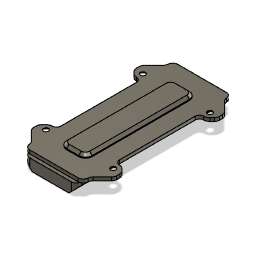
Controller Cooler (P2) [(M)SPPS000000003.2] v2 (Autodesk Fusion 360 design; units mm, degrees)
Autodesk Fusion 360 part; units mm, degrees
sketch "Sketch1" plane through (0, 0, 0) normal (0, 1, 0) x (1, 0, 0)
  line L0 (15.75, 46.1) -> (15.75, -46.1)
  line L1 (-15.75, -46.1) -> (-15.75, 46.1)
  line L2 (-15.75, -46.1) -> (15.75, -46.1)
  line L3 (-15.75, 46.1) -> (15.75, 46.1)
  line L4 (15.25, 45.6) -> (15.25, -45.6)
  line L5 (-15.25, -45.6) -> (15.25, -45.6)
  line L6 (-15.25, -45.6) -> (-15.25, 45.6)
  line L7 (-15.25, 45.6) -> (15.25, 45.6)
  circle A0 centre (19.75, 28.5) radius 3.5
  circle A1 centre (19.75, 28.5) radius 1.5
  circle A2 centre (19.75, -28.5) radius 3.5
  circle A3 centre (19.75, -28.5) radius 1.5
  circle A4 centre (-19.75, 28.5) radius 3.5
  circle A5 centre (-19.75, 28.5) radius 1.5
  circle A6 centre (-19.75, -28.5) radius 3.5
  circle A7 centre (-19.75, -28.5) radius 1.5
  line L8 (-17.25, 47.6) -> (-17.25, 39.6)
  line L9 (-17.25, 39.6) -> (-24.5, 32.35)
  line L10 (-24.5, 28.05) -> (-24.5, 32.35)
  line L11 (-16.9, 20.45) -> (-24.5, 28.05)
  line L12 (-16.9, -20.45) -> (-24.5, -28.05)
  line L13 (-24.5, -28.05) -> (-24.5, -32.35)
  line L14 (-24.5, -32.35) -> (-17.25, -39.6)
  line L15 (-17.25, -39.6) -> (-17.25, -47.6)
  line L16 (17.25, -47.6) -> (17.25, -39.6)
  line L17 (17.25, -39.6) -> (24.5, -32.35)
  line L18 (24.5, -28.05) -> (24.5, -32.35)
  line L19 (16.9, -20.45) -> (24.5, -28.05)
  line L20 (16.9, 20.45) -> (24.5, 28.05)
  line L21 (24.5, 28.05) -> (24.5, 32.35)
  line L22 (24.5, 32.35) -> (17.25, 39.6)
  line L23 (17.25, 39.6) -> (17.25, 47.6)
  line L24 (-17.25, 22.323) -> (-17.25, -22.323)
  line L25 (17.25, -22.323) -> (17.25, 22.323)
  line L26 (-17.25, 47.6) -> (17.25, 47.6)
  line L27 (-17.25, -47.6) -> (17.25, -47.6)
  arc A8 (-22.35, 25.9) -> (-19.75, 24.823) centre (-19.75, 28.5) ccw
  arc A9 (19.75, 24.823) -> (22.35, 25.9) centre (19.75, 28.5) ccw
  arc A10 (-19.75, -24.823) -> (-22.35, -25.9) centre (-19.75, -28.5) ccw
  arc A11 (22.35, -25.9) -> (19.75, -24.823) centre (19.75, -28.5) ccw
  arc A12 (17.25, -22.323) -> (19.75, -24.823) centre (19.75, -22.323) ccw
  arc A13 (-19.75, -24.823) -> (-17.25, -22.323) centre (-19.75, -22.323) ccw
  arc A14 (-17.25, 22.323) -> (-19.75, 24.823) centre (-19.75, 22.323) ccw
  arc A15 (19.75, 24.823) -> (17.25, 22.323) centre (19.75, 22.323) ccw
  dimension "d7" = 31.5
  dimension "d8" = 15.75
  dimension "d99" = -0.5
  dimension "d1586" = 7
  dimension "d1613" = 7
  dimension "d1614" = 7
  dimension "d44" = 7
  dimension "d146" = 3
  dimension "d147" = 3
  dimension "d65" = 3
  dimension "d66" = 3
  dimension "d156" = 1.5
  dimension "d157" = 19.75
  dimension "d158" = 28.5
  dimension "d159" = 28.5
  dimension "d160" = 19.75
  dimension "d161" = 92.2
  dimension "d162" = 46.1
  dimension "d163" = 1.5
  dimension "d164" = 1.5
  dimension "d167" = 1.5
  dimension "d168" = 4.3
  dimension "d169" = 4.3
  dimension "d170" = 4.3
  dimension "d171" = 4.3
  dimension "d172" = 8
  dimension "d173" = 8
  dimension "d174" = 8
  dimension "d175" = 8
  dimension "d176" = 45
  dimension "d177" = 45
  dimension "d178" = 45
  dimension "d179" = 45
  dimension "d180" = 45
  dimension "d181" = 45
  dimension "d182" = 45
  dimension "d183" = 45
  dimension "d185" = 39.5
  dimension "d186" = 4.75
  dimension "d188" = 4.75
  dimension "d197" = 2.5
  dimension "d198" = 2.5
  dimension "d199" = 2.5
  dimension "d200" = 2.5
  constraint vertical L0
  constraint vertical L1
  constraint perpendicular L0 L2
  constraint perpendicular L0 L3
  constraint vertical A2.centre A0.centre
  constraint vertical A4.centre A6.centre
  constraint concentric A4 A5
  constraint concentric A0 A1
  constraint concentric A6 A7
  constraint concentric A2 A3
  constraint horizontal A4.centre A0.centre
  constraint horizontal A2.centre A6.centre
  constraint vertical L10
  constraint vertical L21
  constraint collinear L10 L13
  constraint collinear L18 L21
  constraint collinear L8 L24
  constraint collinear L15 L24
  constraint collinear L16 L25
  constraint collinear L23 L25
  constraint concentric A7 A10
  constraint tangent L12 A10
  constraint concentric A5 A8
  constraint tangent L11 A8
  constraint concentric A3 A11
  constraint tangent L19 A11
  constraint concentric A1 A9
  constraint tangent L20 A9
  constraint coincident L11 A8.start
  constraint coincident L20 A9.end
  constraint coincident L12 A10.end
  constraint coincident L19 A11.start
  constraint tangent A11 A12
  constraint tangent L25 A12
  constraint tangent A10 A13
  constraint tangent L24 A13
  constraint tangent A8 A14
  constraint tangent L24 A14
  constraint tangent A9 A15
  constraint tangent L25 A15
  measures "d7" distance of L0 L1
  measures "d8" distance of origin L1
  measures "d1586" diameter of A2
  measures "d1613" diameter of A0
  measures "d1614" diameter of A6
  measures "d44" diameter of A4
  measures "d146" diameter of A5
  measures "d147" diameter of A1
  measures "d65" diameter of A7
  measures "d66" diameter of A3
  measures "d156" distance of L0 L25
  measures "d157" horizontal distance of origin A4.centre
  measures "d158" vertical distance of origin A4.centre
  measures "d159" vertical distance of origin A6.centre
  measures "d160" horizontal distance of origin A0.centre
  measures "d161" distance of L2 L3
  measures "d162" distance of origin L3
  measures "d163" distance of L3 L26
  measures "d164" distance of L2 L27
  measures "d167" distance of L1 L24
  measures "d168" distance of L20.end L21.end
  measures "d169" distance of L9.end L10.start
  measures "d170" distance of L12.end L13.end
  measures "d171" distance of L17.end L18.start
  measures "d172" distance of L8.end L8.start
  measures "d173" distance of L22.end L23.end
  measures "d174" distance of L16.end L16.start
  measures "d175" distance of L14.end L15.end
  measures "d176" angle of L16 L17
  measures "d177" angle of L19 L25
  measures "d178" angle of L12 L24
  measures "d179" angle of L14 L15
  measures "d180" angle of L8 L9
  measures "d181" angle of L11 L24
  measures "d182" angle of L20 L25
  measures "d183" angle of L22 L23
  measures "d185" distance of A4.centre A0.centre
  measures "d186" distance of A0.centre L21
  measures "d188" distance of A4.centre L10
  measures "d197" radius of A12
  measures "d198" radius of A13
  measures "d199" radius of A14
  measures "d200" radius of A15
extrude "Extrude1" add sketch "Sketch1" against normal blind 2 contours L4 L5 L6 L7
extrude "Extrude2" add sketch "Sketch1" along normal blind 2 contours L0 L1 L2 L3 | L4 L5 L6 L7 | A0 | A2 | A4 | A6 | L8 L9 L10 L11 L12 L13 L14 L15 L16 L17 L18 L19 L20 L21 L22 L23 L24 L25 L26 L27 A8 A9 A10 A11 A12 A13 A14 A15
chamfer "Chamfer1" distance 2 angle 45 4 edges at (18.3515, 0, 27.9576) (18.3515, 0, -29.0424) (-21.1485, 0, -29.0424) (-21.1485, 0, 27.9576)
sketch "Sketch4" plane through (0, -2, 0) normal (0, -1, 0) x (1, 0, 0)
  line L0 (15.75, -45) -> (-15.75, -45)
  line L1 (15.75, -42) -> (-15.75, -42)
  line L2 (15.75, -37) -> (-15.75, -37)
  line L3 (15.75, -44) -> (-15.75, -44)
  line L4 (-15.75, -44) -> (-15.75, -46)
  line L5 (-15.75, -46) -> (15.75, -46)
  line L6 (15.75, -46) -> (15.75, -44)
  line L7 (15.75, -38) -> (-15.75, -38)
  line L8 (-15.75, -38) -> (-15.75, -40)
  line L9 (-15.75, -40) -> (15.75, -40)
  line L10 (15.75, -40) -> (15.75, -38)
  line L11 (15.75, -32) -> (-15.75, -32)
  line L12 (-15.75, -32) -> (-15.75, -34)
  line L13 (-15.75, -34) -> (15.75, -34)
  line L14 (15.75, -34) -> (15.75, -32)
  line L15 (15.75, -26) -> (-15.75, -26)
  line L16 (-15.75, -26) -> (-15.75, -28)
  line L17 (-15.75, -28) -> (15.75, -28)
  line L18 (15.75, -28) -> (15.75, -26)
  line L19 (15.75, -20) -> (-15.75, -20)
  line L20 (-15.75, -20) -> (-15.75, -22)
  line L21 (-15.75, -22) -> (15.75, -22)
  line L22 (15.75, -22) -> (15.75, -20)
  line L23 (15.75, -14) -> (-15.75, -14)
  line L24 (-15.75, -14) -> (-15.75, -16)
  line L25 (-15.75, -16) -> (15.75, -16)
  line L26 (15.75, -16) -> (15.75, -14)
  line L27 (15.75, -8) -> (-15.75, -8)
  line L28 (-15.75, -8) -> (-15.75, -10)
  line L29 (-15.75, -10) -> (15.75, -10)
  line L30 (15.75, -10) -> (15.75, -8)
  line L31 (15.75, -2) -> (-15.75, -2)
  line L32 (-15.75, -2) -> (-15.75, -4)
  line L33 (-15.75, -4) -> (15.75, -4)
  line L34 (15.75, -4) -> (15.75, -2)
  line L35 (15.75, 4) -> (-15.75, 4)
  line L36 (-15.75, 4) -> (-15.75, 2)
  line L37 (-15.75, 2) -> (15.75, 2)
  line L38 (15.75, 2) -> (15.75, 4)
  line L39 (15.75, 10) -> (-15.75, 10)
  line L40 (-15.75, 10) -> (-15.75, 8)
  line L41 (-15.75, 8) -> (15.75, 8)
  line L42 (15.75, 8) -> (15.75, 10)
  line L43 (15.75, 16) -> (-15.75, 16)
  line L44 (-15.75, 16) -> (-15.75, 14)
  line L45 (-15.75, 14) -> (15.75, 14)
  line L46 (15.75, 14) -> (15.75, 16)
  line L47 (15.75, 22) -> (-15.75, 22)
  line L48 (-15.75, 22) -> (-15.75, 20)
  line L49 (-15.75, 20) -> (15.75, 20)
  line L50 (15.75, 20) -> (15.75, 22)
  line L51 (15.75, 28) -> (-15.75, 28)
  line L52 (-15.75, 28) -> (-15.75, 26)
  line L53 (-15.75, 26) -> (15.75, 26)
  line L54 (15.75, 26) -> (15.75, 28)
  line L55 (15.75, 34) -> (-15.75, 34)
  line L56 (-15.75, 34) -> (-15.75, 32)
  line L57 (-15.75, 32) -> (15.75, 32)
  line L58 (15.75, 32) -> (15.75, 34)
  line L59 (15.75, 40) -> (-15.75, 40)
  line L60 (-15.75, 40) -> (-15.75, 38)
  line L61 (-15.75, 38) -> (15.75, 38)
  line L62 (15.75, 38) -> (15.75, 40)
  line L63 (15.75, 46) -> (-15.75, 46)
  line L64 (-15.75, 46) -> (-15.75, 44)
  line L65 (-15.75, 44) -> (15.75, 44)
  line L66 (15.75, 44) -> (15.75, 46)
  line L67 (15.25, 45.6) -> (-15.25, 45.6)
  line L68 (-15.25, 45.6) -> (-15.25, -45.6)
  line L69 (-15.25, -45.6) -> (15.25, -45.6)
  line L70 (15.25, -45.6) -> (15.25, 45.6)
  dimension "d51" = 3
  dimension "d52" = 8
  dimension "d53" = 2
  dimension "d54" = 1
  dimension "d57" = 6
  dimension "d58" = 0
  dimension "d104" = 0.4
  constraint horizontal L2
  constraint horizontal L3
  constraint vertical L4
  constraint horizontal L5
  constraint vertical L6
  measures "d51" distance of L0 L1
  measures "d52" distance of L0 L2
  measures "d53" distance of L3 L5
  measures "d54" distance of L0 L5
  measures "d104" distance of L5 L69
extrude "Extrude5" add sketch "Sketch4" along normal blind 5 contours L0 L68 L69 L70 | L0 L3 L68 L70 | L7 L9 L68 L70 | L11 L13 L68 L70 | L15 L17 L68 L70 | L19 L21 L68 L70 | L23 L25 L68 L70 | L27 L29 L68 L70 | L31 L33 L68 L70 | L35 L37 L68 L70 | L39 L41 L68 L70 | L43 L45 L68 L70 | L47 L49 L68 L70 | L51 L53 L68 L70 | L55 L57 L68 L70 | L59 L61 L68 L70 | L65 L67 L68 L70
chamfer "Chamfer2" distance 0.6 angle 45 32 edges at (0, -7, 34) (0, -7, 32) (0, -7, 28) (0, -7, 26) (0, -7, 22) (0, -7, 20) (0, -7, 16) (0, -7, 14) (0, -7, 10) (0, -7, 8) (0, -7, 4) (0, -7, 2) (0, -7, -2) (0, -7, -4) (0, -7, -8) (0, -7, -10) (0, -7, -14) (0, -7, -16) (0, -7, -20) (0, -7, -22) (0, -7, -26) (0, -7, -28) (0, -7, -32) (0, -7, -34) (0, -7, -38) (0, -7, -40) (0, -7, -44) (0, -7, 40) (0, -7, 38) (0, -7, 44) (0, -7, -45.6) (0, -7, 45.6)
chamfer "Chamfer3" distance 5 angle 45 32 edges at (-15.25, -7, 39) (-15.25, -7, 44.8) (-15.25, -7, 33) (-15.25, -7, 27) (-15.25, -7, 21) (-15.25, -7, 15) (-15.25, -7, 9) (-15.25, -7, 3) (-15.25, -7, -3) (-15.25, -7, -9) (-15.25, -7, -15) (-15.25, -7, -21) (-15.25, -7, -27) (-15.25, -7, -44.8) (-15.25, -7, -39) (-15.25, -7, -33) (15.25, -7, -44.8) (15.25, -7, -39) (15.25, -7, -33) (15.25, -7, -27) (15.25, -7, -21) (15.25, -7, -15) (15.25, -7, -9) (15.25, -7, -3) (15.25, -7, 3) (15.25, -7, 9) (15.25, -7, 15) (15.25, -7, 21) (15.25, -7, 27) (15.25, -7, 33) (15.25, -7, 39) (15.25, -7, 44.8)
fillet "Fillet1" radius 3 16 edges at (17.25, 1, 39.6) (24.5, 1, 32.35) (24.5, 1, 28.05) (24.5, 1, -28.05) (17.25, 1, -39.6) (24.5, 1, -32.35) (-17.25, 1, -39.6) (-24.5, 1, -32.35) (-24.5, 1, -28.05) (-24.5, 1, 28.05) (-24.5, 1, 32.35) (-17.25, 1, 39.6) (-17.25, 1, 47.6) (17.25, 1, 47.6) (-17.25, 1, -47.6) (17.25, 1, -47.6)
sketch "Sketch5" plane through (0, 2, 0) normal (0, 1, 0) x (-1, 0, 0)
  line L0 (9.45, -35.5) -> (16.45, -35.5)
  line L1 (9.45, -35.5) -> (9.45, -29)
  line L2 (9.45, -29) -> (16.45, -29)
  line L3 (16.45, -29) -> (16.45, -35.5)
  circle A0 centre (10.4182, -33.75) radius 2
  circle A1 centre (10.4182, -30.75) radius 2
  line L4 (8.4182, -33.75) -> (8.4182, -30.75)
  line L5 (10.4182, -35.75) -> (16.45, -35.75)
  line L6 (16.45, -35.75) -> (16.45, -35.5)
  line L7 (10.4182, -28.75) -> (16.45, -28.75)
  line L8 (16.45, -28.75) -> (16.45, -29)
  line L9 (10.4182, -36.75) -> (17.45, -36.75)
  line L10 (17.45, -36.75) -> (17.45, -35.5)
  circle A2 centre (10.4182, -33.75) radius 3
  line L11 (7.4182, -33.75) -> (7.4182, -30.75)
  circle A3 centre (10.4182, -30.75) radius 3
  line L12 (10.4182, -27.75) -> (17.45, -27.75)
  line L13 (17.45, -27.75) -> (17.45, -29)
  line L14 (-22.35, -25.9) -> (-23.6213, -27.1713)
  line L15 (-24.5, -29.2926) -> (-24.5, -31.1074)
  line L16 (-23.6213, -33.2287) -> (-18.1287, -38.7213)
  line L17 (-17.25, -40.8426) -> (-17.25, -44.6)
  line L18 (17.25, -44.6) -> (17.25, -40.8426)
  line L19 (18.1287, -38.7213) -> (23.6213, -33.2287)
  line L20 (24.5, -31.1074) -> (24.5, -29.2926)
  line L21 (23.6213, -27.1713) -> (22.35, -25.9)
  line L22 (17.25, -22.323) -> (17.25, 22.323)
  line L23 (22.35, 25.9) -> (23.6213, 27.1713)
  line L24 (24.5, 29.2926) -> (24.5, 31.1074)
  line L25 (23.6213, 33.2287) -> (18.1287, 38.7213)
  line L26 (17.25, 40.8426) -> (17.25, 44.6)
  line L27 (-17.25, 44.6) -> (-17.25, 40.8426)
  line L28 (-18.1287, 38.7213) -> (-23.6213, 33.2287)
  line L29 (-24.5, 31.1074) -> (-24.5, 29.2926)
  line L30 (-23.6213, 27.1713) -> (-22.35, 25.9)
  circle A4 centre (-19.75, -28.5) radius 1.5
  circle A5 centre (19.75, -28.5) radius 1.5
  circle A6 centre (-19.75, 28.5) radius 1.5
  circle A7 centre (19.75, 28.5) radius 1.5
  arc A8 (24.5, 31.1074) -> (23.6213, 33.2287) centre (21.5, 31.1074) ccw
  arc A9 (17.25, 40.8426) -> (18.1287, 38.7213) centre (20.25, 40.8426) ccw
  arc A10 (-18.1287, 38.7213) -> (-17.25, 40.8426) centre (-20.25, 40.8426) ccw
  arc A11 (-23.6213, 33.2287) -> (-24.5, 31.1074) centre (-21.5, 31.1074) ccw
  arc A12 (-24.5, 29.2926) -> (-23.6213, 27.1713) centre (-21.5, 29.2926) ccw
  arc A13 (-23.6213, -27.1713) -> (-24.5, -29.2926) centre (-21.5, -29.2926) ccw
  arc A14 (-24.5, -31.1074) -> (-23.6213, -33.2287) centre (-21.5, -31.1074) ccw
  arc A15 (-17.25, -40.8426) -> (-18.1287, -38.7213) centre (-20.25, -40.8426) ccw
  arc A16 (18.1287, -38.7213) -> (17.25, -40.8426) centre (20.25, -40.8426) ccw
  arc A17 (23.6213, -33.2287) -> (24.5, -31.1074) centre (21.5, -31.1074) ccw
  arc A18 (24.5, -29.2926) -> (23.6213, -27.1713) centre (21.5, -29.2926) ccw
  arc A19 (23.6213, 27.1713) -> (24.5, 29.2926) centre (21.5, 29.2926) ccw
  line L31 (14.25, 47.6) -> (-14.25, 47.6)
  line L32 (-14.25, -47.6) -> (14.25, -47.6)
  arc A20 (-17.25, -44.6) -> (-14.25, -47.6) centre (-14.25, -44.6) ccw
  arc A21 (14.25, -47.6) -> (17.25, -44.6) centre (14.25, -44.6) ccw
  arc A22 (17.25, 44.6) -> (14.25, 47.6) centre (14.25, 44.6) ccw
  arc A23 (-14.25, 47.6) -> (-17.25, 44.6) centre (-14.25, 44.6) ccw
  line L33 (-17.25, 22.323) -> (-17.25, -22.323)
  arc A24 (22.35, -25.9) -> (19.75, -24.823) centre (19.75, -28.5) ccw
  arc A25 (17.25, -22.323) -> (19.75, -24.823) centre (19.75, -22.323) ccw
  arc A26 (19.75, 24.823) -> (17.25, 22.323) centre (19.75, 22.323) ccw
  arc A27 (19.75, 24.823) -> (22.35, 25.9) centre (19.75, 28.5) ccw
  arc A28 (-22.35, 25.9) -> (-19.75, 24.823) centre (-19.75, 28.5) ccw
  arc A29 (-17.25, 22.323) -> (-19.75, 24.823) centre (-19.75, 22.323) ccw
  arc A30 (-19.75, -24.823) -> (-17.25, -22.323) centre (-19.75, -22.323) ccw
  arc A31 (-19.75, -24.823) -> (-22.35, -25.9) centre (-19.75, -28.5) ccw
  dimension "d140" = 4
  dimension "d141" = 4
  dimension "d142" = 3
  dimension "d111" = 6.5
  dimension "d115" = 1
  dimension "d116" = 1
  dimension "d117" = -1
  dimension "d118" = 1
  dimension "d119" = -1
  constraint perpendicular L2 L3
  constraint perpendicular L1 L2
  constraint perpendicular L0 L3
  constraint vertical A0.centre A1.centre
  constraint coincident L1.end A1
  constraint coincident L0.start A0
  constraint coincident A0 L4.start
  constraint coincident A1 L4.end
  constraint tangent A1 L4
  constraint parallel L1 L4
  constraint coincident A0 L5.start
  constraint tangent A0 L5
  constraint coincident A1 L7.start
  constraint tangent A1 L7
  measures "d140" diameter of A1
  measures "d141" diameter of A0
  measures "d142" distance of A0.centre A1.centre
  measures "d111" distance of L0 L2
sketch "Sketch6" plane through (0, 2, 0) normal (0, 1, 0) x (-1, 0, 0)
  arc A0 (-17.25, -44.6) -> (-14.25, -47.6) centre (-14.25, -44.6) ccw
  line L0 (-14.25, -47.6) -> (14.25, -47.6)
  arc A1 (14.25, -47.6) -> (17.25, -44.6) centre (14.25, -44.6) ccw
  line L1 (17.25, -44.6) -> (17.25, -40.8426)
  arc A2 (18.1287, -38.7213) -> (17.25, -40.8426) centre (20.25, -40.8426) ccw
  line L2 (18.1287, -38.7213) -> (23.6213, -33.2287)
  arc A3 (23.6213, -33.2287) -> (24.5, -31.1074) centre (21.5, -31.1074) ccw
  line L3 (24.5, -31.1074) -> (24.5, -29.2926)
  arc A4 (24.5, -29.2926) -> (23.6213, -27.1713) centre (21.5, -29.2926) ccw
  line L4 (23.6213, -27.1713) -> (22.35, -25.9)
  line L5 (17.25, -22.323) -> (17.25, 22.323)
  line L6 (22.35, 25.9) -> (23.6213, 27.1713)
  arc A5 (23.6213, 27.1713) -> (24.5, 29.2926) centre (21.5, 29.2926) ccw
  line L7 (24.5, 29.2926) -> (24.5, 31.1074)
  arc A6 (24.5, 31.1074) -> (23.6213, 33.2287) centre (21.5, 31.1074) ccw
  line L8 (23.6213, 33.2287) -> (18.1287, 38.7213)
  arc A7 (17.25, 40.8426) -> (18.1287, 38.7213) centre (20.25, 40.8426) ccw
  line L9 (17.25, 40.8426) -> (17.25, 44.6)
  arc A8 (17.25, 44.6) -> (14.25, 47.6) centre (14.25, 44.6) ccw
  line L10 (14.25, 47.6) -> (-14.25, 47.6)
  arc A9 (-14.25, 47.6) -> (-17.25, 44.6) centre (-14.25, 44.6) ccw
  line L11 (-17.25, 44.6) -> (-17.25, 40.8426)
  arc A10 (-18.1287, 38.7213) -> (-17.25, 40.8426) centre (-20.25, 40.8426) ccw
  line L12 (-18.1287, 38.7213) -> (-23.6213, 33.2287)
  arc A11 (-23.6213, 33.2287) -> (-24.5, 31.1074) centre (-21.5, 31.1074) ccw
  line L13 (-24.5, 31.1074) -> (-24.5, 29.2926)
  arc A12 (-24.5, 29.2926) -> (-23.6213, 27.1713) centre (-21.5, 29.2926) ccw
  line L14 (-23.6213, 27.1713) -> (-22.35, 25.9)
  line L15 (-17.25, 22.323) -> (-17.25, -22.323)
  line L16 (-22.35, -25.9) -> (-23.6213, -27.1713)
  arc A13 (-23.6213, -27.1713) -> (-24.5, -29.2926) centre (-21.5, -29.2926) ccw
  line L17 (-24.5, -29.2926) -> (-24.5, -31.1074)
  arc A14 (-24.5, -31.1074) -> (-23.6213, -33.2287) centre (-21.5, -31.1074) ccw
  line L18 (-23.6213, -33.2287) -> (-18.1287, -38.7213)
  arc A15 (-17.25, -40.8426) -> (-18.1287, -38.7213) centre (-20.25, -40.8426) ccw
  line L19 (-17.25, -40.8426) -> (-17.25, -44.6)
  circle A16 centre (-19.75, 28.5) radius 1.5
  circle A17 centre (19.75, 28.5) radius 1.5
  circle A18 centre (-19.75, -28.5) radius 1.5
  circle A19 centre (19.75, -28.5) radius 1.5
  line L20 (3.55, -32.6) -> (-3.55, -32.6)
  line L21 (-7.55, -28.6) -> (-7.55, 28.6)
  line L22 (-3.55, 32.6) -> (3.55, 32.6)
  line L23 (7.55, 28.6) -> (7.55, -28.6)
  arc A20 (3.55, -32.6) -> (7.55, -28.6) centre (3.55, -28.6) ccw
  arc A21 (-7.55, -28.6) -> (-3.55, -32.6) centre (-3.55, -28.6) ccw
  arc A22 (-3.55, 32.6) -> (-7.55, 28.6) centre (-3.55, 28.6) ccw
  arc A23 (7.55, 28.6) -> (3.55, 32.6) centre (3.55, 28.6) ccw
  arc A24 (22.35, -25.9) -> (19.75, -24.823) centre (19.75, -28.5) ccw
  arc A25 (17.25, -22.323) -> (19.75, -24.823) centre (19.75, -22.323) ccw
  arc A26 (19.75, 24.823) -> (17.25, 22.323) centre (19.75, 22.323) ccw
  arc A27 (19.75, 24.823) -> (22.35, 25.9) centre (19.75, 28.5) ccw
  arc A28 (-22.35, 25.9) -> (-19.75, 24.823) centre (-19.75, 28.5) ccw
  arc A29 (-17.25, 22.323) -> (-19.75, 24.823) centre (-19.75, 22.323) ccw
  arc A30 (-19.75, -24.823) -> (-17.25, -22.323) centre (-19.75, -22.323) ccw
  arc A31 (-19.75, -24.823) -> (-22.35, -25.9) centre (-19.75, -28.5) ccw
  dimension "d189" = 9.7
  dimension "d190" = 9.7
  dimension "d191" = 15
  dimension "d192" = 15
  dimension "d193" = 4
  constraint horizontal L20
  constraint vertical L21
  constraint horizontal L22
  constraint vertical L23
  constraint tangent L20 A20
  constraint tangent L23 A20
  constraint tangent L20 A21
  constraint tangent L21 A21
  constraint equal A20 A21
  constraint tangent L21 A22
  constraint tangent L22 A22
  constraint equal A20 A22
  constraint tangent L22 A23
  constraint tangent L23 A23
  constraint equal A20 A23
  measures "d189" distance of L5 L23
  measures "d190" distance of L15 L21
  measures "d191" distance of L0 L20
  measures "d192" distance of L10 L22
  measures "d193" radius of A20
extrude "Extrude8" add sketch "Sketch6" along normal blind 2 contours L20 L21 L22 L23 A20 A21 A22 A23
chamfer "Chamfer5" distance 1.5 angle 45 8 edges at (-7.55, 4, 0) (-6.3784, 4, 31.4284) (0, 4, 32.6) (6.3784, 4, 31.4284) (7.55, 4, 0) (6.3784, 4, -31.4284) (0, 4, -32.6) (-6.3784, 4, -31.4284)
sketch "Sketch7" plane through (0, 2, 0) normal (0, 1, 0) x (-1, 0, 0)
  line L0 (3.55, -32.6) -> (-3.55, -32.6)
  arc A0 (-7.55, -28.6) -> (-3.55, -32.6) centre (-3.55, -28.6) ccw
  line L1 (-7.55, -28.6) -> (-7.55, 28.6)
  arc A1 (-3.55, 32.6) -> (-7.55, 28.6) centre (-3.55, 28.6) ccw
  line L2 (-3.55, 32.6) -> (3.55, 32.6)
  arc A2 (7.55, 28.6) -> (3.55, 32.6) centre (3.55, 28.6) ccw
  line L3 (7.55, 28.6) -> (7.55, -28.6)
  arc A3 (3.55, -32.6) -> (7.55, -28.6) centre (3.55, -28.6) ccw
  arc A4 (-17.25, -44.6) -> (-14.25, -47.6) centre (-14.25, -44.6) ccw
  line L4 (-14.25, -47.6) -> (14.25, -47.6)
  arc A5 (14.25, -47.6) -> (17.25, -44.6) centre (14.25, -44.6) ccw
  line L5 (17.25, -44.6) -> (17.25, -40.8426)
  arc A6 (18.1287, -38.7213) -> (17.25, -40.8426) centre (20.25, -40.8426) ccw
  line L6 (18.1287, -38.7213) -> (23.6213, -33.2287)
  arc A7 (23.6213, -33.2287) -> (24.5, -31.1074) centre (21.5, -31.1074) ccw
  line L7 (24.5, -31.1074) -> (24.5, -29.2926)
  arc A8 (24.5, -29.2926) -> (23.6213, -27.1713) centre (21.5, -29.2926) ccw
  line L8 (23.6213, -27.1713) -> (22.35, -25.9)
  arc A9 (22.35, -25.9) -> (19.75, -24.823) centre (19.75, -28.5) ccw
  arc A10 (17.25, -22.323) -> (19.75, -24.823) centre (19.75, -22.323) ccw
  line L9 (17.25, -22.323) -> (17.25, 22.323)
  arc A11 (19.75, 24.823) -> (17.25, 22.323) centre (19.75, 22.323) ccw
  arc A12 (19.75, 24.823) -> (22.35, 25.9) centre (19.75, 28.5) ccw
  line L10 (22.35, 25.9) -> (23.6213, 27.1713)
  arc A13 (23.6213, 27.1713) -> (24.5, 29.2926) centre (21.5, 29.2926) ccw
  line L11 (24.5, 29.2926) -> (24.5, 31.1074)
  arc A14 (24.5, 31.1074) -> (23.6213, 33.2287) centre (21.5, 31.1074) ccw
  line L12 (23.6213, 33.2287) -> (18.1287, 38.7213)
  arc A15 (17.25, 40.8426) -> (18.1287, 38.7213) centre (20.25, 40.8426) ccw
  line L13 (17.25, 40.8426) -> (17.25, 44.6)
  arc A16 (17.25, 44.6) -> (14.25, 47.6) centre (14.25, 44.6) ccw
  line L14 (14.25, 47.6) -> (-14.25, 47.6)
  arc A17 (-14.25, 47.6) -> (-17.25, 44.6) centre (-14.25, 44.6) ccw
  line L15 (-17.25, 44.6) -> (-17.25, 40.8426)
  arc A18 (-18.1287, 38.7213) -> (-17.25, 40.8426) centre (-20.25, 40.8426) ccw
  line L16 (-18.1287, 38.7213) -> (-23.6213, 33.2287)
  arc A19 (-23.6213, 33.2287) -> (-24.5, 31.1074) centre (-21.5, 31.1074) ccw
  line L17 (-24.5, 31.1074) -> (-24.5, 29.2926)
  arc A20 (-24.5, 29.2926) -> (-23.6213, 27.1713) centre (-21.5, 29.2926) ccw
  line L18 (-23.6213, 27.1713) -> (-22.35, 25.9)
  arc A21 (-22.35, 25.9) -> (-19.75, 24.823) centre (-19.75, 28.5) ccw
  arc A22 (-17.25, 22.323) -> (-19.75, 24.823) centre (-19.75, 22.323) ccw
  line L19 (-17.25, 22.323) -> (-17.25, -22.323)
  arc A23 (-19.75, -24.823) -> (-17.25, -22.323) centre (-19.75, -22.323) ccw
  arc A24 (-19.75, -24.823) -> (-22.35, -25.9) centre (-19.75, -28.5) ccw
  line L20 (-22.35, -25.9) -> (-23.6213, -27.1713)
  arc A25 (-23.6213, -27.1713) -> (-24.5, -29.2926) centre (-21.5, -29.2926) ccw
  line L21 (-24.5, -29.2926) -> (-24.5, -31.1074)
  arc A26 (-24.5, -31.1074) -> (-23.6213, -33.2287) centre (-21.5, -31.1074) ccw
  line L22 (-23.6213, -33.2287) -> (-18.1287, -38.7213)
  arc A27 (-17.25, -40.8426) -> (-18.1287, -38.7213) centre (-20.25, -40.8426) ccw
  line L23 (-17.25, -40.8426) -> (-17.25, -44.6)
  circle A28 centre (19.75, -28.5) radius 1.5
  circle A29 centre (19.75, 28.5) radius 1.5
  circle A30 centre (-19.75, 28.5) radius 1.5
  circle A31 centre (-19.75, -28.5) radius 1.5
  line L24 (14.2549, 43.6) -> (-14.2549, 43.6)
  arc A32 (17.2549, 40.6) -> (14.2549, 43.6) centre (14.2549, 40.6) ccw
  arc A33 (-14.2549, 43.6) -> (-17.2549, 40.6) centre (-14.2549, 40.6) ccw
  line L25 (-14.2549, -43.6) -> (14.2549, -43.6)
  arc A34 (14.2549, -43.6) -> (17.2549, -40.6) centre (14.2549, -40.6) ccw
  arc A35 (-17.2549, -40.6) -> (-14.2549, -43.6) centre (-14.2549, -40.6) ccw
  dimension "d205" = 3
  dimension "d206" = 3
  dimension "d207" = 4
  dimension "d211" = 3
  dimension "d212" = 3
  dimension "d213" = 4
  constraint parallel L14 L24
  constraint tangent L24 A32
  constraint tangent L24 A33
  constraint parallel L4 L25
  constraint tangent L25 A34
  constraint tangent L25 A35
  constraint tangent A6 A34
  constraint tangent A27 A35
  constraint tangent A15 A32
  constraint tangent A18 A33
  measures "d205" radius of A32
  measures "d206" radius of A33
  measures "d207" distance of L14 L24
  measures "d211" radius of A34
  measures "d212" radius of A35
  measures "d213" distance of L4 L25
extrude "Extrude9" cut sketch "Sketch7" against normal blind 2 contours A4 L4 A5 L5 A6 A27 L23 L25 A34 A35 | A15 L13 A16 L14 A17 L15 A18 L24 A32 A33
fillet "Fillet2" radius 3 4 edges at (15.25, -1, 45.6) (-15.25, -1, 45.6) (15.25, -1, -45.6) (-15.25, -1, -45.6)
equation "d8 = d7 / 2"
equation "d162 = d161 / 2"
